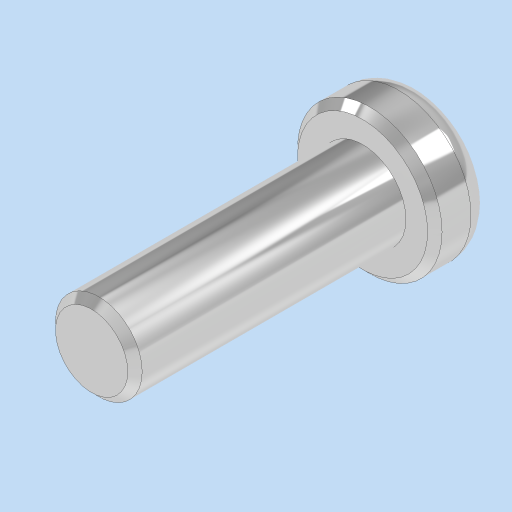
# Autodesk Inventor part: pan_head_screw_M1.2x4
Saved by Autodesk Inventor 2024 (Build 280153000, 153)
## iProperties
Created: 2025-05-11
Part Number: pan_head_screw_M1.2x4
Material: Nickel-Copper Alloy 400
Document SubType Name: Modeling
Designer: XxPan
Density: 8.83 g/cm^3
Appearance: Chrome - Polished
Author: XxPan
Autodesk Inventor part; units mm, degrees
ref_plane "YZ Plane" through (0, 0, 0) normal (1, 0, 0) x (0, 1, 0)
ref_plane "XZ Plane" through (0, 0, 0) normal (0, 1, 0) x (-1, 0, 0)
ref_plane "XY Plane" through (0, 0, 0) normal (0, 0, 1) x (1, 0, 0)
sketch "Sketch1" plane through (0, 0, 0) normal (0, 0, 1) x (1, 0, 0)
  circle A0 centre (0, 0) radius 1
  dimension "d0" = 2
  constraints: 1 centre point, 1 coincident
  measures "d0" diameter of A0
extrude "Extrusion1" add sketch "Sketch1" against normal blind 0.8
sketch "Sketch2" plane through (0, 0, 0) normal (0, 0, 1) x (1, 0, 0)
  circle A0 centre (0, 0) radius 1 projected
  circle A1 centre (0, 0) radius 0.6
  dimension "d3" = 1.2
  constraints: 1 centre point, 1 coincident
  measures "d3" diameter of A1
extrude "Extrusion2" add sketch "Sketch2" along normal blind 3.75 contours A1
fillet "Fillet1" radius 0.3 1 edges at (-1, 0, -0.8)
chamfer "Chamfer1" distance 0.1 angle 45 2 edges at (-1, 0, 0) (-0.6, 0, 3.75)
sketch "Sketch3" plane through (0, 0, -0.8) normal (0, 0, -1) x (-1, 0, 0)
  line L0 (-0.15, 0.15) -> (-0.15, 0.6)
  line L1 (-0.15, 0.6) -> (0.15, 0.6)
  line L2 (0.15, 0.6) -> (0.15, 0.15)
  line L3 (0.15, 0.15) -> (0.6, 0.15)
  line L4 (0.6, 0.15) -> (0.6, -0.15)
  line L5 (0.6, -0.15) -> (0.15, -0.15)
  line L6 (0.15, -0.15) -> (0.15, -0.6)
  line L7 (0.15, -0.6) -> (-0.15, -0.6)
  line L8 (-0.15, -0.6) -> (-0.15, -0.15)
  line L9 (-0.15, -0.15) -> (-0.6, -0.15)
  line L10 (-0.6, -0.15) -> (-0.6, 0.15)
  line L11 (-0.6, 0.15) -> (-0.15, 0.15)
  line L12 (1.4, 0) -> (-1.4, 0) construction
  line L13 (0, -1.4) -> (0, 1.4) construction
  point P0 (0, 0)
  dimension "d10" = 1.2
  dimension "d11" = 0.3
  constraints: 24 end point, 4 collinear, 4 equal length, 4 perpendicular, 3 horizontal, 3 parallel, 2 vertical, 2 other
  measures "d10" distance between parallel lines of L4 L10
  measures "d11" distance of L0.end L1.end
extrude "Extrusion3" cut sketch "Sketch3" against normal blind 0.5
body "Solid1"
